Autodesk Inventor part; units mm, degrees
(part 2 of 2)
  line L161 (52.6404, 40.6164) -> (52.6404, 40.3516)
  line L162 (52.6404, 40.3516) -> (50.5162, 40.3516)
  line L163 (50.5162, 40.3516) -> (52.6404, 39.7455)
  line L164 (52.6404, 39.7455) -> (52.6404, 39.4984)
  line L165 (52.6404, 39.4984) -> (50.4789, 38.8943)
  line L166 (50.4789, 38.8943) -> (52.6404, 38.8943)
  line L167 (52.6404, 38.8943) -> (52.6404, 38.6295)
  line L168 (52.6404, 41.8638) -> (50.1004, 41.8638)
  line L169 (50.1004, 41.8638) -> (50.1004, 42.1384)
  line L170 (50.1004, 42.1384) -> (51.3596, 42.1384)
  line L171 (51.3596, 42.1384) -> (50.1004, 43.174)
  line L172 (50.1004, 43.174) -> (50.1004, 43.5487)
  line L173 (50.1004, 43.5487) -> (51.1301, 42.6739)
  line L174 (51.1301, 42.6739) -> (52.6404, 43.5859)
  line L175 (52.6404, 43.5859) -> (52.6404, 43.2211)
  line L176 (52.6404, 43.2211) -> (51.3576, 42.4797)
  line L177 (51.3576, 42.4797) -> (51.7597, 42.1384)
  line L178 (51.7597, 42.1384) -> (52.6404, 42.1384)
  line L179 (52.6404, 42.1384) -> (52.6404, 41.8638)
  line L180 (52.05, 44.8059) -> (52.0892, 45.0687)
  spline S97 degree 2 poles (52.0892, 45.0687) (52.3834, 45.0021) (52.6835, 44.6588) (52.6835, 44.4038) knots 0 0 0 1 2 2 2
  spline S98 degree 2 poles (52.6835, 44.4038) (52.6835, 44.0841) (52.1971, 43.6879) (51.7362, 43.6879) knots 0 0 0 1 2 2 2
  spline S99 degree 2 poles (51.7362, 43.6879) (51.2595, 43.6879) (50.7594, 44.088) (50.7594, 44.394) knots 0 0 0 1 2 2 2
  spline S100 degree 2 poles (50.7594, 44.394) (50.7594, 44.6863) (51.2517, 45.0785) (51.7185, 45.0785) knots 0 0 0 1 2 2 2
  line L181 (51.7185, 45.0785) -> (51.8009, 45.0766)
  line L182 (51.8009, 45.0766) -> (51.8009, 43.9507)
  spline S101 degree 2 poles (51.8009, 43.9507) (52.1108, 43.9664) (52.4266, 44.2234) (52.4266, 44.4058) knots 0 0 0 1 2 2 2
  spline S102 degree 2 poles (52.4266, 44.4058) (52.4266, 44.6941) (52.05, 44.8059) knots 0 0 0 1 1 1
  line L183 (51.5439, 43.9664) -> (51.5439, 44.8079)
  spline S103 degree 2 poles (51.5439, 44.8079) (51.3047, 44.7902) (51.187, 44.7059) knots 0 0 0 1 1 1
  spline S104 degree 2 poles (51.187, 44.7059) (51.0163, 44.5823) (51.0163, 44.3921) knots 0 0 0 1 1 1
  spline S105 degree 2 poles (51.0163, 44.3921) (51.0163, 44.2214) (51.3027, 43.9782) (51.5439, 43.9664) knots 0 0 0 1 2 2 2
  line L184 (53.3504, 45.3865) -> (53.0562, 45.359)
  spline S106 degree 2 poles (53.0562, 45.359) (53.0836, 45.4434) (53.0836, 45.5042) knots 0 0 0 1 1 1
  spline S107 degree 2 poles (53.0836, 45.5042) (53.0836, 45.5846) (53.0169, 45.6905) (52.9483, 45.7238) knots 0 0 0 1 2 2 2
  spline S108 degree 2 poles (52.9483, 45.7238) (52.9248, 45.7356) (52.6384, 45.8239) knots 0 0 0 1 1 1
  line L185 (52.6384, 45.8239) -> (50.8006, 45.2531)
  line L186 (50.8006, 45.2531) -> (50.8006, 45.5277)
  line L187 (50.8006, 45.5277) -> (51.8617, 45.8435)
  spline S109 degree 2 poles (51.8617, 45.8435) (52.0598, 45.9004) (52.2853, 45.9514) knots 0 0 0 1 1 1
  spline S110 degree 2 poles (52.2853, 45.9514) (52.0716, 45.9945) (51.8695, 46.0553) knots 0 0 0 1 1 1
  line L188 (51.8695, 46.0553) -> (50.8006, 46.377)
  line L189 (50.8006, 46.377) -> (50.8006, 46.6339)
  line L190 (50.8006, 46.6339) -> (52.6717, 46.0612)
  spline S111 degree 2 poles (52.6717, 46.0612) (53.0366, 45.9494) (53.2798, 45.82) (53.3876, 45.6552) (53.3876, 45.5512) knots 0 0 0 1 2 3 3 3
  spline S112 degree 2 poles (53.3876, 45.5512) (53.3876, 45.4787) (53.3504, 45.3865) knots 0 0 0 1 1 1
  point P0 (0, 0)
  constraints: 2 horizontal, 1 vertical, 6 other
sketch "Sketch15" plane through (0, 4.35, 0) normal (0, 1, 0) x (1, 0, 0)
  point P0 (0, 0)
sketch "Sketch16" plane through (0, 1.6, 0) normal (0, 1, 0) x (1, 0, 0)
  line L0 (10.625, 36) -> (13.125, 36)
  line L1 (13.125, 36) -> (13.125, 40.5)
  line L2 (13.125, 40.5) -> (10.625, 40.5)
  line L3 (10.625, 40.5) -> (10.625, 36)
  line L4 (23.75, 43.5) -> (32.75, 43.5) projected
  line L5 (6.5, 7.1) -> (6.5, 57.9) projected
  line L6 (17.25, 61) -> (17.25, 23) projected
  point P0 (0, 0)
  dimension "d172" = 3
  dimension "d173" = 2.5
  dimension "d174" = 4.5
  dimension "d175" = 4.125
  dimension "d176" = 4.125
  constraints: 8 end point, 2 parallel, 1 horizontal, 1 perpendicular
  measures "d172" distance between parallel lines of L4 L2
  measures "d173" distance of L1.end L2.end
  measures "d174" distance of L0.end L1.end
  measures "d175" distance between parallel lines of L5 L3
  measures "d176" distance between parallel lines of L6 L1
extrude "Extrusion17" add sketch "Sketch16" along normal blind 1
ref_plane "Work Plane1" through (13.125, 1.6, -39.6) normal (0, 0, -1) x (-1, 0, 0)
sketch "Sketch17" plane through (13.125, 1.6, -39.6) normal (0, 0, -1) x (-1, 0, 0)
  line L0 (0, 0) -> (0, 1) projected
  line L1 (0, 0.9) -> (-0.25, 0.9)
  line L2 (0, 0.8) -> (-0.25, 0.8)
  arc A0 (-0.25, 0.8) -> (-1.05, 0) centre (-0.25, 0) ccw
  arc A1 (-0.25, 0.9) -> (-1.15, 0.1) centre (-0.25, -0.0062) ccw
  line L3 (-1.05, 0) -> (-1.5, 0)
  line L4 (-1.5, 0) -> (-1.5, 0.1)
  line L5 (-1.5, 0.1) -> (-1.15, 0.1)
  line L6 (0, 0.8) -> (0, 0.9)
  point P0 (13.125, -1.6)
  dimension "d180" = 0.1
  dimension "d181" = 0.1
  dimension "d182" = 1.5
  dimension "d183" = 0.25
  dimension "d184" = 0.1
  dimension "d185" = 0.1
  constraints: 12 end point, 4 point on circle, 3 perpendicular, 2 centre point, 2 horizontal, 2 point on line, 2 tangent, 1 collinear, 1 horizontal alignment, 1 line through centre, 1 vertical alignment
  measures "d180" distance between parallel lines of L1 L2
  measures "d181" distance of L3.end L4.end
  measures "d182" distance between parallel lines of L0 L4
  measures "d183" distance of L2.start L2.end
  measures "d184" horizontal distance of L3.start L5.end
  measures "d185" distance of L0.end L1.start
extrude "Extrusion18" add sketch "Sketch17" along normal mid plane 0.25
ref_plane "Work Plane2" through (13.125, 1.6, -39.15) normal (0, 0, -1) x (-1, 0, 0)
mirror "Mirror1" about plane through (13.125, 1.6, -39.15) normal (0, 0, -1) of "Extrusion18"
ref_plane "Work Plane3" through (13.125, 1.6, -38.25) normal (0, 0, -1) x (-1, 0, 0)
mirror "Mirror2" about plane through (13.125, 1.6, -38.25) normal (0, 0, -1) of "Extrusion18", "Mirror1"
ref_plane "Work Plane4" through (11.875, 1.6, -36) normal (1, 0, 0) x (0, 0, -1)
mirror "Mirror3" about plane through (11.875, 1.6, -36) normal (1, 0, 0) of "Extrusion18", "Mirror1", "Mirror2"
sketch "Sketch18" plane through (0, 1.6, 0) normal (0, 1, 0) x (1, 0, 0)
  line L0 (6.5, 7.1) -> (6.5, 57.9) projected
  line L1 (6.5, 8.69) -> (7.5, 8.69)
  line L2 (7.5, 8.69) -> (7.5, 8.05)
  line L3 (7.5, 8.05) -> (6.5, 8.05)
  line L4 (6.5, 8.05) -> (6.5, 8.69)
  line L5 (5.55, 48.69) -> (4.91, 48.69) projected
  line L6 (4.91, 48.69) -> (4.91, 49.33) projected
  line L7 (4.91, 49.33) -> (5.55, 49.33) projected
  line L8 (5.55, 49.33) -> (5.55, 48.69) projected
  line L9 (5.55, 38.53) -> (4.91, 38.53) projected
  line L10 (4.91, 38.53) -> (4.91, 39.17) projected
  line L11 (4.91, 39.17) -> (5.55, 39.17) projected
  line L12 (5.55, 39.17) -> (5.55, 38.53) projected
  line L13 (3.09, 56.31) -> (2.45, 56.31) projected
  line L14 (2.45, 56.31) -> (2.45, 56.95) projected
  line L15 (2.45, 56.95) -> (3.09, 56.95) projected
  line L16 (3.09, 56.95) -> (3.09, 56.31) projected
  line L17 (5.55, 10.59) -> (4.91, 10.59) projected
  line L18 (4.91, 10.59) -> (4.91, 11.23) projected
  line L19 (4.91, 11.23) -> (5.55, 11.23) projected
  line L20 (5.55, 11.23) -> (5.55, 10.59) projected
  line L21 (3.09, 13.13) -> (2.45, 13.13) projected
  line L22 (2.45, 13.13) -> (2.45, 13.77) projected
  line L23 (2.45, 13.77) -> (3.09, 13.77) projected
  line L24 (3.09, 13.77) -> (3.09, 13.13) projected
  line L25 (3.09, 46.15) -> (2.45, 46.15) projected
  line L26 (2.45, 46.15) -> (2.45, 46.79) projected
  line L27 (2.45, 46.79) -> (3.09, 46.79) projected
  line L28 (3.09, 46.79) -> (3.09, 46.15) projected
  line L29 (3.09, 23.29) -> (2.45, 23.29) projected
  line L30 (2.45, 23.29) -> (2.45, 23.93) projected
  line L31 (2.45, 23.93) -> (3.09, 23.93) projected
  line L32 (3.09, 23.93) -> (3.09, 23.29) projected
  line L33 (3.09, 20.75) -> (2.45, 20.75) projected
  line L34 (2.45, 20.75) -> (2.45, 21.39) projected
  line L35 (2.45, 21.39) -> (3.09, 21.39) projected
  line L36 (3.09, 21.39) -> (3.09, 20.75) projected
  line L37 (3.09, 28.37) -> (2.45, 28.37) projected
  line L38 (2.45, 28.37) -> (2.45, 29.01) projected
  line L39 (2.45, 29.01) -> (3.09, 29.01) projected
  line L40 (3.09, 29.01) -> (3.09, 28.37) projected
  line L41 (3.09, 33.45) -> (2.45, 33.45) projected
  line L42 (2.45, 33.45) -> (2.45, 34.09) projected
  line L43 (2.45, 34.09) -> (3.09, 34.09) projected
  line L44 (3.09, 34.09) -> (3.09, 33.45) projected
  line L45 (3.09, 30.91) -> (2.45, 30.91) projected
  line L46 (2.45, 30.91) -> (2.45, 31.55) projected
  line L47 (2.45, 31.55) -> (3.09, 31.55) projected
  line L48 (3.09, 31.55) -> (3.09, 30.91) projected
  line L49 (5.55, 25.83) -> (4.91, 25.83) projected
  line L50 (4.91, 25.83) -> (4.91, 26.47) projected
  line L51 (4.91, 26.47) -> (5.55, 26.47) projected
  line L52 (5.55, 26.47) -> (5.55, 25.83) projected
  line L53 (5.55, 23.29) -> (4.91, 23.29) projected
  line L54 (4.91, 23.29) -> (4.91, 23.93) projected
  line L55 (4.91, 23.93) -> (5.55, 23.93) projected
  line L56 (5.55, 23.93) -> (5.55, 23.29) projected
  line L57 (5.55, 20.75) -> (4.91, 20.75) projected
  line L58 (4.91, 20.75) -> (4.91, 21.39) projected
  line L59 (4.91, 21.39) -> (5.55, 21.39) projected
  line L60 (5.55, 21.39) -> (5.55, 20.75) projected
  line L61 (3.09, 18.21) -> (2.45, 18.21) projected
  line L62 (2.45, 18.21) -> (2.45, 18.85) projected
  line L63 (2.45, 18.85) -> (3.09, 18.85) projected
  line L64 (3.09, 18.85) -> (3.09, 18.21) projected
  line L65 (3.09, 15.67) -> (2.45, 15.67) projected
  line L66 (2.45, 15.67) -> (2.45, 16.31) projected
  line L67 (2.45, 16.31) -> (3.09, 16.31) projected
  line L68 (3.09, 16.31) -> (3.09, 15.67) projected
  line L69 (3.09, 53.77) -> (2.45, 53.77) projected
  line L70 (2.45, 53.77) -> (2.45, 54.41) projected
  line L71 (2.45, 54.41) -> (3.09, 54.41) projected
  line L72 (3.09, 54.41) -> (3.09, 53.77) projected
  line L73 (5.55, 56.31) -> (4.91, 56.31) projected
  line L74 (4.91, 56.31) -> (4.91, 56.95) projected
  line L75 (4.91, 56.95) -> (5.55, 56.95) projected
  line L76 (5.55, 56.95) -> (5.55, 56.31) projected
  line L77 (5.55, 41.07) -> (4.91, 41.07) projected
  line L78 (4.91, 41.07) -> (4.91, 41.71) projected
  line L79 (4.91, 41.71) -> (5.55, 41.71) projected
  line L80 (5.55, 41.71) -> (5.55, 41.07) projected
  line L81 (5.55, 51.23) -> (4.91, 51.23) projected
  line L82 (4.91, 51.23) -> (4.91, 51.87) projected
  line L83 (4.91, 51.87) -> (5.55, 51.87) projected
  line L84 (5.55, 51.87) -> (5.55, 51.23) projected
  line L85 (5.55, 46.15) -> (4.91, 46.15) projected
  line L86 (4.91, 46.15) -> (4.91, 46.79) projected
  line L87 (4.91, 46.79) -> (5.55, 46.79) projected
  line L88 (5.55, 46.79) -> (5.55, 46.15) projected
  line L89 (5.55, 35.99) -> (4.91, 35.99) projected
  line L90 (4.91, 35.99) -> (4.91, 36.63) projected
  line L91 (4.91, 36.63) -> (5.55, 36.63) projected
  line L92 (5.55, 36.63) -> (5.55, 35.99) projected
  line L93 (5.55, 8.05) -> (4.91, 8.05) projected
  line L94 (4.91, 8.05) -> (4.91, 8.69) projected
  line L95 (4.91, 8.69) -> (5.55, 8.69) projected
  line L96 (5.55, 8.69) -> (5.55, 8.05) projected
  line L97 (3.09, 51.23) -> (2.45, 51.23) projected
  line L98 (2.45, 51.23) -> (2.45, 51.87) projected
  line L99 (2.45, 51.87) -> (3.09, 51.87) projected
  line L100 (3.09, 51.87) -> (3.09, 51.23) projected
  line L101 (3.09, 48.69) -> (2.45, 48.69) projected
  line L102 (2.45, 48.69) -> (2.45, 49.33) projected
  line L103 (2.45, 49.33) -> (3.09, 49.33) projected
  line L104 (3.09, 49.33) -> (3.09, 48.69) projected
  line L105 (5.55, 18.21) -> (4.91, 18.21) projected
  line L106 (4.91, 18.21) -> (4.91, 18.85) projected
  line L107 (4.91, 18.85) -> (5.55, 18.85) projected
  line L108 (5.55, 18.85) -> (5.55, 18.21) projected
  line L109 (3.09, 41.07) -> (2.45, 41.07) projected
  line L110 (2.45, 41.07) -> (2.45, 41.71) projected
  line L111 (2.45, 41.71) -> (3.09, 41.71) projected
  line L112 (3.09, 41.71) -> (3.09, 41.07) projected
  line L113 (3.09, 25.83) -> (2.45, 25.83) projected
  line L114 (2.45, 25.83) -> (2.45, 26.47) projected
  line L115 (2.45, 26.47) -> (3.09, 26.47) projected
  line L116 (3.09, 26.47) -> (3.09, 25.83) projected
  line L117 (3.09, 35.99) -> (2.45, 35.99) projected
  line L118 (2.45, 35.99) -> (2.45, 36.63) projected
  line L119 (2.45, 36.63) -> (3.09, 36.63) projected
  line L120 (3.09, 36.63) -> (3.09, 35.99) projected
  line L121 (5.55, 30.91) -> (4.91, 30.91) projected
  line L122 (4.91, 30.91) -> (4.91, 31.55) projected
  line L123 (4.91, 31.55) -> (5.55, 31.55) projected
  line L124 (5.55, 31.55) -> (5.55, 30.91) projected
  line L125 (5.55, 28.37) -> (4.91, 28.37) projected
  line L126 (4.91, 28.37) -> (4.91, 29.01) projected
  line L127 (4.91, 29.01) -> (5.55, 29.01) projected
  line L128 (5.55, 29.01) -> (5.55, 28.37) projected
  line L129 (3.09, 38.53) -> (2.45, 38.53) projected
  line L130 (2.45, 38.53) -> (2.45, 39.17) projected
  line L131 (2.45, 39.17) -> (3.09, 39.17) projected
  line L132 (3.09, 39.17) -> (3.09, 38.53) projected
  line L133 (3.09, 8.69) -> (3.09, 8.05) projected
  line L134 (3.09, 8.05) -> (2.45, 8.05) projected
  line L135 (2.45, 8.05) -> (2.45, 8.69) projected
  line L136 (2.45, 8.69) -> (3.09, 8.69) projected
  line L137 (3.09, 43.61) -> (2.45, 43.61) projected
  line L138 (2.45, 43.61) -> (2.45, 44.25) projected
  line L139 (2.45, 44.25) -> (3.09, 44.25) projected
  line L140 (3.09, 44.25) -> (3.09, 43.61) projected
  line L141 (5.55, 15.67) -> (4.91, 15.67) projected
  line L142 (4.91, 15.67) -> (4.91, 16.31) projected
  line L143 (4.91, 16.31) -> (5.55, 16.31) projected
  line L144 (5.55, 16.31) -> (5.55, 15.67) projected
  line L145 (5.55, 13.13) -> (4.91, 13.13) projected
  line L146 (4.91, 13.13) -> (4.91, 13.77) projected
  line L147 (4.91, 13.77) -> (5.55, 13.77) projected
  line L148 (5.55, 13.77) -> (5.55, 13.13) projected
  line L149 (3.09, 10.59) -> (2.45, 10.59) projected
  line L150 (2.45, 10.59) -> (2.45, 11.23) projected
  line L151 (2.45, 11.23) -> (3.09, 11.23) projected
  line L152 (3.09, 11.23) -> (3.09, 10.59) projected
  line L153 (5.55, 33.45) -> (4.91, 33.45) projected
  line L154 (4.91, 33.45) -> (4.91, 34.09) projected
  line L155 (4.91, 34.09) -> (5.55, 34.09) projected
  line L156 (5.55, 34.09) -> (5.55, 33.45) projected
  line L157 (5.55, 43.61) -> (4.91, 43.61) projected
  line L158 (4.91, 43.61) -> (4.91, 44.25) projected
  line L159 (4.91, 44.25) -> (5.55, 44.25) projected
  line L160 (5.55, 44.25) -> (5.55, 43.61) projected
  line L161 (5.55, 53.77) -> (4.91, 53.77) projected
  line L162 (4.91, 53.77) -> (4.91, 54.41) projected
  line L163 (4.91, 54.41) -> (5.55, 54.41) projected
  line L164 (5.55, 54.41) -> (5.55, 53.77) projected
  line L165 (6.5, 7.1) -> (6.5, 57.9) projected
  line L166 (6.5, 57.9) -> (1.5, 57.9) projected
  line L167 (1.5, 57.9) -> (1.5, 7.1) projected
  line L168 (1.5, 7.1) -> (6.5, 7.1) projected
  line L169 (6.5, 11.23) -> (7.5, 11.23)
  line L170 (7.5, 10.59) -> (6.5, 10.59)
  line L171 (7.5, 11.23) -> (7.5, 10.59)
  line L172 (6.5, 10.59) -> (6.5, 11.23)
  line L173 (6.5, 13.77) -> (7.5, 13.77)
  line L174 (7.5, 13.13) -> (6.5, 13.13)
  line L175 (7.5, 13.77) -> (7.5, 13.13)
  line L176 (6.5, 13.13) -> (6.5, 13.77)
  line L177 (6.5, 16.31) -> (7.5, 16.31)
  line L178 (7.5, 15.67) -> (6.5, 15.67)
  line L179 (7.5, 16.31) -> (7.5, 15.67)
  line L180 (6.5, 15.67) -> (6.5, 16.31)
  line L181 (6.5, 18.85) -> (7.5, 18.85)
  line L182 (7.5, 18.21) -> (6.5, 18.21)
  line L183 (7.5, 18.85) -> (7.5, 18.21)
  line L184 (6.5, 18.21) -> (6.5, 18.85)
  line L185 (6.5, 21.39) -> (7.5, 21.39)
  line L186 (7.5, 20.75) -> (6.5, 20.75)
  line L187 (7.5, 21.39) -> (7.5, 20.75)
  line L188 (6.5, 20.75) -> (6.5, 21.39)
  line L189 (6.5, 23.93) -> (7.5, 23.93)
  line L190 (7.5, 23.29) -> (6.5, 23.29)
  line L191 (7.5, 23.93) -> (7.5, 23.29)
  line L192 (6.5, 23.29) -> (6.5, 23.93)
  line L193 (6.5, 26.47) -> (7.5, 26.47)
  line L194 (7.5, 25.83) -> (6.5, 25.83)
  line L195 (7.5, 26.47) -> (7.5, 25.83)
  line L196 (6.5, 25.83) -> (6.5, 26.47)
  line L197 (6.5, 29.01) -> (7.5, 29.01)
  line L198 (7.5, 28.37) -> (6.5, 28.37)
  line L199 (7.5, 29.01) -> (7.5, 28.37)
  line L200 (6.5, 28.37) -> (6.5, 29.01)
  line L201 (6.5, 31.55) -> (7.5, 31.55)
  line L202 (7.5, 30.91) -> (6.5, 30.91)
  line L203 (7.5, 31.55) -> (7.5, 30.91)
  line L204 (6.5, 30.91) -> (6.5, 31.55)
  line L205 (6.5, 34.09) -> (7.5, 34.09)
  line L206 (7.5, 33.45) -> (6.5, 33.45)
  line L207 (7.5, 34.09) -> (7.5, 33.45)
  line L208 (6.5, 33.45) -> (6.5, 34.09)
  line L209 (6.5, 36.63) -> (7.5, 36.63)
  line L210 (7.5, 35.99) -> (6.5, 35.99)
  line L211 (7.5, 36.63) -> (7.5, 35.99)
  line L212 (6.5, 35.99) -> (6.5, 36.63)
  line L213 (6.5, 39.17) -> (7.5, 39.17)
  line L214 (7.5, 38.53) -> (6.5, 38.53)
  line L215 (7.5, 39.17) -> (7.5, 38.53)
  line L216 (6.5, 38.53) -> (6.5, 39.17)
  line L217 (6.5, 41.71) -> (7.5, 41.71)
  line L218 (7.5, 41.07) -> (6.5, 41.07)
  line L219 (7.5, 41.71) -> (7.5, 41.07)
  line L220 (6.5, 41.07) -> (6.5, 41.71)
  line L221 (6.5, 44.25) -> (7.5, 44.25)
  line L222 (7.5, 43.61) -> (6.5, 43.61)
  line L223 (7.5, 44.25) -> (7.5, 43.61)
  line L224 (6.5, 43.61) -> (6.5, 44.25)
  line L225 (6.5, 46.79) -> (7.5, 46.79)
  line L226 (7.5, 46.15) -> (6.5, 46.15)
  line L227 (7.5, 46.79) -> (7.5, 46.15)
  line L228 (6.5, 46.15) -> (6.5, 46.79)
  line L229 (6.5, 49.33) -> (7.5, 49.33)
  line L230 (7.5, 48.69) -> (6.5, 48.69)
  line L231 (7.5, 49.33) -> (7.5, 48.69)
  line L232 (6.5, 48.69) -> (6.5, 49.33)
  line L233 (6.5, 51.87) -> (7.5, 51.87)
  line L234 (7.5, 51.23) -> (6.5, 51.23)
  line L235 (7.5, 51.87) -> (7.5, 51.23)
  line L236 (6.5, 51.23) -> (6.5, 51.87)
  line L237 (6.5, 54.41) -> (7.5, 54.41)
  line L238 (7.5, 53.77) -> (6.5, 53.77)
  line L239 (7.5, 54.41) -> (7.5, 53.77)
  line L240 (6.5, 53.77) -> (6.5, 54.41)
  line L241 (6.5, 56.95) -> (7.5, 56.95)
  line L242 (7.5, 56.31) -> (6.5, 56.31)
  line L243 (7.5, 56.95) -> (7.5, 56.31)
  line L244 (6.5, 56.31) -> (6.5, 56.95)
  point P0 (0, 0)
  point P1 (6.5, 56.95)
  point P2 (6.5, 56.31)
  point P3 (6.5, 54.41)
  point P4 (6.5, 53.77)
  point P5 (6.5, 51.87)
  point P6 (6.5, 51.23)
  point P7 (6.5, 49.33)
  point P8 (6.5, 48.69)
  point P9 (6.5, 46.79)
  point P10 (6.5, 46.15)
  point P11 (6.5, 44.25)
  point P12 (6.5, 43.61)
  point P13 (6.5, 41.71)
  point P14 (6.5, 41.07)
  point P15 (6.5, 39.17)
  point P16 (6.5, 38.53)
  point P17 (6.5, 36.63)
  point P18 (6.5, 35.99)
  point P19 (6.5, 34.09)
  point P20 (6.5, 33.45)
  point P21 (6.5, 31.55)
  point P22 (6.5, 30.91)
  point P23 (6.5, 29.01)
  point P24 (6.5, 28.37)
  point P25 (6.5, 26.47)
  point P26 (6.5, 25.83)
  point P27 (6.5, 23.93)
  point P28 (6.5, 23.29)
  point P29 (6.5, 21.39)
  point P30 (6.5, 20.75)
  point P31 (6.5, 18.85)
  point P32 (6.5, 18.21)
  point P33 (6.5, 16.31)
  point P34 (6.5, 15.67)
  point P35 (6.5, 13.77)
  point P36 (6.5, 13.13)
  point P37 (6.5, 11.23)
  dimension "d190" = 1
  dimension "d193" = 2.54
  constraints: 160 end point, 76 vertical alignment, 40 parallel, 38 collinear, 3 horizontal alignment, 1 horizontal, 1 perpendicular, 1 point on line, 2 other
  measures "d190" distance of L2.end L3.end
  measures "d193" distance of L1.start L169.start
extrude "Extrusion19" add sketch "Sketch18" along normal blind 0.25 contours L0 L1 L2 L3 | L0 L169 L171 L170 | L241 L243 L242 L0 | L0 L173 L175 L174 | L237 L239 L238 L0 | L0 L177 L179 L178 | L233 L235 L234 L0 | L0 L181 L183 L182 | L229 L231 L230 L0 | L0 L185 L187 L186 | L225 L227 L226 L0 | L0 L189 L191 L190 | L221 L223 L222 L0 | L0 L193 L195 L194 | L217 L219 L218 L0 | L0 L197 L199 L198 | L213 L215 L214 L0 | L0 L201 L203 L202 | L209 L211 L210 L0 | L0 L205 L207 L206
ref_plane "Work Plane5" through (4, 1.6, -57.9) normal (1, 0, 0) x (0, 0, -1)
mirror "Mirror4" about plane through (4, 1.6, -57.9) normal (1, 0, 0) of "Extrusion19"
extrude "Extrusion20" add sketch "Sketch14" along normal blind 0.01
sketch "Sketch19" plane through (0, 0, 0) normal (0, -1, 0) x (1, 0, 0)
  circle A0 centre (53, -3.5) radius 3 projected
  circle A1 centre (4, -3.5) radius 3 projected
  circle A2 centre (53, -61.5) radius 3 projected
  circle A3 centre (4, -61.5) radius 3 projected
  point P0 (0, 0)
extrude "Extrusion21" cut sketch "Sketch19" against normal blind 0.02
sketch "Sketch20" plane through (0, 0, 0) normal (0, -1, 0) x (1, 0, 0)
  line L0 (5.55, -48.69) -> (4.91, -48.69) projected
  line L1 (4.91, -48.69) -> (4.91, -49.33) projected
  line L2 (4.91, -49.33) -> (5.55, -49.33) projected
  line L3 (5.55, -49.33) -> (5.55, -48.69) projected
  line L4 (5.55, -38.53) -> (4.91, -38.53) projected
  line L5 (4.91, -38.53) -> (4.91, -39.17) projected
  line L6 (4.91, -39.17) -> (5.55, -39.17) projected
  line L7 (5.55, -39.17) -> (5.55, -38.53) projected
  line L8 (3.09, -56.31) -> (2.45, -56.31) projected
  line L9 (2.45, -56.31) -> (2.45, -56.95) projected
  line L10 (2.45, -56.95) -> (3.09, -56.95) projected
  line L11 (3.09, -56.95) -> (3.09, -56.31) projected
  line L12 (5.55, -10.59) -> (4.91, -10.59) projected
  line L13 (4.91, -10.59) -> (4.91, -11.23) projected
  line L14 (4.91, -11.23) -> (5.55, -11.23) projected
  line L15 (5.55, -11.23) -> (5.55, -10.59) projected
  line L16 (3.09, -13.13) -> (2.45, -13.13) projected
  line L17 (2.45, -13.13) -> (2.45, -13.77) projected
  line L18 (2.45, -13.77) -> (3.09, -13.77) projected
  line L19 (3.09, -13.77) -> (3.09, -13.13) projected
  line L20 (3.09, -46.15) -> (2.45, -46.15) projected
  line L21 (2.45, -46.15) -> (2.45, -46.79) projected
  line L22 (2.45, -46.79) -> (3.09, -46.79) projected
  line L23 (3.09, -46.79) -> (3.09, -46.15) projected
  line L24 (3.09, -23.29) -> (2.45, -23.29) projected
  line L25 (2.45, -23.29) -> (2.45, -23.93) projected
  line L26 (2.45, -23.93) -> (3.09, -23.93) projected
  line L27 (3.09, -23.93) -> (3.09, -23.29) projected
  line L28 (3.09, -20.75) -> (2.45, -20.75) projected
  line L29 (2.45, -20.75) -> (2.45, -21.39) projected
  line L30 (2.45, -21.39) -> (3.09, -21.39) projected
  line L31 (3.09, -21.39) -> (3.09, -20.75) projected
  line L32 (3.09, -28.37) -> (2.45, -28.37) projected
  line L33 (2.45, -28.37) -> (2.45, -29.01) projected
  line L34 (2.45, -29.01) -> (3.09, -29.01) projected
  line L35 (3.09, -29.01) -> (3.09, -28.37) projected
  line L36 (3.09, -33.45) -> (2.45, -33.45) projected
  line L37 (2.45, -33.45) -> (2.45, -34.09) projected
  line L38 (2.45, -34.09) -> (3.09, -34.09) projected
  line L39 (3.09, -34.09) -> (3.09, -33.45) projected
  line L40 (3.09, -30.91) -> (2.45, -30.91) projected
  line L41 (2.45, -30.91) -> (2.45, -31.55) projected
  line L42 (2.45, -31.55) -> (3.09, -31.55) projected
  line L43 (3.09, -31.55) -> (3.09, -30.91) projected
  line L44 (5.55, -25.83) -> (4.91, -25.83) projected
  line L45 (4.91, -25.83) -> (4.91, -26.47) projected
  line L46 (4.91, -26.47) -> (5.55, -26.47) projected
  line L47 (5.55, -26.47) -> (5.55, -25.83) projected
  line L48 (5.55, -23.29) -> (4.91, -23.29) projected
  line L49 (4.91, -23.29) -> (4.91, -23.93) projected
  line L50 (4.91, -23.93) -> (5.55, -23.93) projected
  line L51 (5.55, -23.93) -> (5.55, -23.29) projected
  line L52 (5.55, -20.75) -> (4.91, -20.75) projected
  line L53 (4.91, -20.75) -> (4.91, -21.39) projected
  line L54 (4.91, -21.39) -> (5.55, -21.39) projected
  line L55 (5.55, -21.39) -> (5.55, -20.75) projected
  line L56 (3.09, -18.21) -> (2.45, -18.21) projected
  line L57 (2.45, -18.21) -> (2.45, -18.85) projected
  line L58 (2.45, -18.85) -> (3.09, -18.85) projected
  line L59 (3.09, -18.85) -> (3.09, -18.21) projected
  line L60 (3.09, -15.67) -> (2.45, -15.67) projected
  line L61 (2.45, -15.67) -> (2.45, -16.31) projected
  line L62 (2.45, -16.31) -> (3.09, -16.31) projected
  line L63 (3.09, -16.31) -> (3.09, -15.67) projected
  line L64 (3.09, -53.77) -> (2.45, -53.77) projected
  line L65 (2.45, -53.77) -> (2.45, -54.41) projected
  line L66 (2.45, -54.41) -> (3.09, -54.41) projected
  line L67 (3.09, -54.41) -> (3.09, -53.77) projected
  line L68 (5.55, -56.31) -> (4.91, -56.31) projected
  line L69 (4.91, -56.31) -> (4.91, -56.95) projected
  line L70 (4.91, -56.95) -> (5.55, -56.95) projected
  line L71 (5.55, -56.95) -> (5.55, -56.31) projected
  line L72 (5.55, -41.07) -> (4.91, -41.07) projected
  line L73 (4.91, -41.07) -> (4.91, -41.71) projected
  line L74 (4.91, -41.71) -> (5.55, -41.71) projected
  line L75 (5.55, -41.71) -> (5.55, -41.07) projected
  line L76 (5.55, -51.23) -> (4.91, -51.23) projected
  line L77 (4.91, -51.23) -> (4.91, -51.87) projected
  line L78 (4.91, -51.87) -> (5.55, -51.87) projected
  line L79 (5.55, -51.87) -> (5.55, -51.23) projected
  line L80 (5.55, -46.15) -> (4.91, -46.15) projected
  line L81 (4.91, -46.15) -> (4.91, -46.79) projected
  line L82 (4.91, -46.79) -> (5.55, -46.79) projected
  line L83 (5.55, -46.79) -> (5.55, -46.15) projected
  line L84 (5.55, -35.99) -> (4.91, -35.99) projected
  line L85 (4.91, -35.99) -> (4.91, -36.63) projected
  line L86 (4.91, -36.63) -> (5.55, -36.63) projected
  line L87 (5.55, -36.63) -> (5.55, -35.99) projected
  line L88 (5.55, -8.05) -> (4.91, -8.05) projected
  line L89 (4.91, -8.05) -> (4.91, -8.69) projected
  line L90 (4.91, -8.69) -> (5.55, -8.69) projected
  line L91 (5.55, -8.69) -> (5.55, -8.05) projected
  line L92 (3.09, -51.23) -> (2.45, -51.23) projected
  line L93 (2.45, -51.23) -> (2.45, -51.87) projected
  line L94 (2.45, -51.87) -> (3.09, -51.87) projected
  line L95 (3.09, -51.87) -> (3.09, -51.23) projected
  line L96 (3.09, -48.69) -> (2.45, -48.69) projected
  line L97 (2.45, -48.69) -> (2.45, -49.33) projected
  line L98 (2.45, -49.33) -> (3.09, -49.33) projected
  line L99 (3.09, -49.33) -> (3.09, -48.69) projected
  line L100 (5.55, -18.21) -> (4.91, -18.21) projected
  line L101 (4.91, -18.21) -> (4.91, -18.85) projected
  line L102 (4.91, -18.85) -> (5.55, -18.85) projected
  line L103 (5.55, -18.85) -> (5.55, -18.21) projected
  line L104 (3.09, -41.07) -> (2.45, -41.07) projected
  line L105 (2.45, -41.07) -> (2.45, -41.71) projected
  line L106 (2.45, -41.71) -> (3.09, -41.71) projected
  line L107 (3.09, -41.71) -> (3.09, -41.07) projected
  line L108 (3.09, -25.83) -> (2.45, -25.83) projected
  line L109 (2.45, -25.83) -> (2.45, -26.47) projected
  line L110 (2.45, -26.47) -> (3.09, -26.47) projected
  line L111 (3.09, -26.47) -> (3.09, -25.83) projected
  line L112 (3.09, -35.99) -> (2.45, -35.99) projected
  line L113 (2.45, -35.99) -> (2.45, -36.63) projected
  line L114 (2.45, -36.63) -> (3.09, -36.63) projected
  line L115 (3.09, -36.63) -> (3.09, -35.99) projected
  line L116 (5.55, -30.91) -> (4.91, -30.91) projected
  line L117 (4.91, -30.91) -> (4.91, -31.55) projected
  line L118 (4.91, -31.55) -> (5.55, -31.55) projected
  line L119 (5.55, -31.55) -> (5.55, -30.91) projected
  line L120 (5.55, -28.37) -> (4.91, -28.37) projected
  line L121 (4.91, -28.37) -> (4.91, -29.01) projected
  line L122 (4.91, -29.01) -> (5.55, -29.01) projected
  line L123 (5.55, -29.01) -> (5.55, -28.37) projected
  line L124 (3.09, -38.53) -> (2.45, -38.53) projected
  line L125 (2.45, -38.53) -> (2.45, -39.17) projected
  line L126 (2.45, -39.17) -> (3.09, -39.17) projected
  line L127 (3.09, -39.17) -> (3.09, -38.53) projected
  line L128 (3.09, -8.69) -> (3.09, -8.05) projected
  line L129 (3.09, -8.05) -> (2.45, -8.05) projected
  line L130 (2.45, -8.05) -> (2.45, -8.69) projected
  line L131 (2.45, -8.69) -> (3.09, -8.69) projected
  line L132 (3.09, -43.61) -> (2.45, -43.61) projected
  line L133 (2.45, -43.61) -> (2.45, -44.25) projected
  line L134 (2.45, -44.25) -> (3.09, -44.25) projected
  line L135 (3.09, -44.25) -> (3.09, -43.61) projected
  line L136 (5.55, -15.67) -> (4.91, -15.67) projected
  line L137 (4.91, -15.67) -> (4.91, -16.31) projected
  line L138 (4.91, -16.31) -> (5.55, -16.31) projected
  line L139 (5.55, -16.31) -> (5.55, -15.67) projected
  line L140 (5.55, -13.13) -> (4.91, -13.13) projected
  line L141 (4.91, -13.13) -> (4.91, -13.77) projected
  line L142 (4.91, -13.77) -> (5.55, -13.77) projected
  line L143 (5.55, -13.77) -> (5.55, -13.13) projected
  line L144 (3.09, -10.59) -> (2.45, -10.59) projected
  line L145 (2.45, -10.59) -> (2.45, -11.23) projected
  line L146 (2.45, -11.23) -> (3.09, -11.23) projected
  line L147 (3.09, -11.23) -> (3.09, -10.59) projected
  line L148 (5.55, -33.45) -> (4.91, -33.45) projected
  line L149 (4.91, -33.45) -> (4.91, -34.09) projected
  line L150 (4.91, -34.09) -> (5.55, -34.09) projected
  line L151 (5.55, -34.09) -> (5.55, -33.45) projected
  line L152 (5.55, -43.61) -> (4.91, -43.61) projected
  line L153 (4.91, -43.61) -> (4.91, -44.25) projected
  line L154 (4.91, -44.25) -> (5.55, -44.25) projected
  line L155 (5.55, -44.25) -> (5.55, -43.61) projected
  line L156 (5.55, -53.77) -> (4.91, -53.77) projected
  line L157 (4.91, -53.77) -> (4.91, -54.41) projected
  line L158 (4.91, -54.41) -> (5.55, -54.41) projected
  line L159 (5.55, -54.41) -> (5.55, -53.77) projected
  line L160 (6.5, -7.1) -> (6.5, -57.9) projected
  line L161 (6.5, -57.9) -> (1.5, -57.9) projected
  line L162 (1.5, -57.9) -> (1.5, -7.1) projected
  line L163 (1.5, -7.1) -> (6.5, -7.1) projected
  point P0 (0, 0)
extrude "Extrusion22" cut sketch "Sketch20" against normal through all contours L3 L2 L1 L0 | L7 L6 L5 L4 | L11 L10 L9 L8 | L15 L14 L13 L12 | L19 L18 L17 L16 | L23 L22 L21 L20 | L27 L26 L25 L24 | L31 L30 L29 L28 | L35 L34 L33 L32 | L39 L38 L37 L36 | L43 L42 L41 L40 | L47 L46 L45 L44 | L51 L50 L49 L48 | L55 L54 L53 L52 | L59 L58 L57 L56 | L63 L62 L61 L60 | L67 L66 L65 L64 | L71 L70 L69 L68 | L75 L74 L73 L72 | L79 L78 L77 L76 | L83 L82 L81 L80 | L87 L86 L85 L84 | L91 L90 L89 L88 | L95 L94 L93 L92 | L99 L98 L97 L96 | L103 L102 L101 L100 | L107 L106 L105 L104 | L111 L110 L109 L108 | L115 L114 L113 L112 | L119 L118 L117 L116 | L123 L122 L121 L120 | L127 L126 L125 L124 | L131 L130 L129 L128 | L135 L134 L133 L132 | L139 L138 L137 L136 | L143 L142 L141 L140 | L147 L146 L145 L144 | L151 L150 L149 L148 | L155 L154 L153 L152 | L159 L158 L157 L156
extrude "Extrusion23" add sketch "Sketch11" along normal blind 1.9 contours L0 L7 L2 L8
sketch "Sketch21" plane through (0, 1.6, 0) normal (0, 1, 0) x (1, 0, 0)
  line L0 (45.3625, 29.5277) -> (48.4125, 29.5277)
  line L1 (48.9125, 30.0277) -> (48.9125, 45.7978)
  line L2 (48.4125, 46.2978) -> (45.3625, 46.2978)
  line L3 (44.8625, 45.7978) -> (44.8625, 30.0277)
  arc A0 (44.8625, 30.0277) -> (45.3625, 29.5277) centre (45.3625, 30.0277) ccw
  arc A1 (48.4125, 29.5277) -> (48.9125, 30.0277) centre (48.4125, 30.0277) ccw
  arc A2 (48.9125, 45.7978) -> (48.4125, 46.2978) centre (48.4125, 45.7978) ccw
  arc A3 (45.3625, 46.2978) -> (44.8625, 45.7978) centre (45.3625, 45.7978) ccw
  line L4 (44.6125, 30.0277) -> (44.6125, 45.7978)
  arc A4 (45.3625, 46.5478) -> (44.6125, 45.7978) centre (45.3625, 45.7978) ccw
  line L5 (45.3625, 46.5478) -> (48.4125, 46.5478)
  arc A5 (49.1625, 45.7978) -> (48.4125, 46.5478) centre (48.4125, 45.7978) ccw
  line L6 (49.1625, 45.7978) -> (49.1625, 30.0277)
  arc A6 (48.4125, 29.2777) -> (49.1625, 30.0277) centre (48.4125, 30.0277) ccw
  line L7 (48.4125, 29.2777) -> (45.3625, 29.2777)
  arc A7 (44.6125, 30.0277) -> (45.3625, 29.2777) centre (45.3625, 30.0277) ccw
  line L8 (55.5, 47.5) -> (41, 47.5) projected
  line L9 (56.5, 3.5) -> (56.5, 46.5) projected
  line L10 (48.4125, 42.5313) -> (48.4125, 42.861) projected
  line L11 (45.3625, 43.69) -> (45.3625, 41.707) projected
  line L12 (45.3625, 30.2277) -> (48.4125, 30.2277) projected
  line L13 (47.0841, 45.5978) -> (46.7356, 45.5978) projected
  point P0 (0, 0)
  dimension "d211" = 0.5
  dimension "d212" = 0.25
  dimension "d215" = 0.5
  dimension "d216" = 0.5
  dimension "d217" = 0.7
  dimension "d218" = 0.7
  constraints: 16 end point, 16 point on circle, 8 centre point, 8 tangent, 4 parallel, 3 equal radius, 2 perpendicular, 1 horizontal, 7 other
  measures "d211" radius of A0
  measures "d212" distance between parallel lines of L4 L3
  measures "d215" distance between parallel lines of L10 L1
  measures "d216" distance between parallel lines of L3 L11
  measures "d217" distance between parallel lines of L0 L12
  measures "d218" distance between parallel lines of L13 L2
extrude "Extrusion24" add sketch "Sketch21" along normal up to surface (0.01 mm away)
sketch "Sketch22" plane through (0, 4.35, 0) normal (0, 1, 0) x (1, 0, 0)
  line L0 (30.75, 34.6545) -> (25.75, 34.6545) construction
  line L1 (25.75, 34.6545) -> (25.75, 37.1545) construction
  line L2 (25.75, 37.1545) -> (30.75, 37.1545) construction
  line L3 (30.75, 37.1545) -> (30.75, 34.6545) construction
  line L4 (26.4257, 37.1545) -> (31.4257, 37.1545) construction
  line L5 (31.4257, 37.1545) -> (31.4257, 34.6545) construction
  line L6 (31.4257, 34.6545) -> (26.4257, 34.6545) construction
  line L7 (26.4257, 34.6545) -> (26.4257, 37.1545) construction
  line L8 (23.4045, 33.5) -> (23.4045, 42.5) projected
  line L9 (33.0955, 42.5) -> (33.0955, 33.5) projected
  line L10 (32.75, 33.1545) -> (23.75, 33.1545) projected
  line L11 (30.4788, 36.3941) -> (30.4788, 35.3941)
  line L12 (30.4788, 35.3941) -> (30.3202, 35.3941)
  line L13 (30.3202, 35.3941) -> (30.3202, 35.805)
  line L14 (30.3202, 35.805) -> (29.6975, 35.805)
  line L15 (29.6975, 35.805) -> (29.6975, 35.3941)
  line L16 (29.6975, 35.3941) -> (29.539, 35.3941)
  line L17 (29.539, 35.3941) -> (29.539, 36.3941)
  line L18 (29.539, 36.3941) -> (29.6975, 36.3941)
  line L19 (29.6975, 36.3941) -> (29.6975, 35.9231)
  line L20 (29.6975, 35.9231) -> (30.3202, 35.9231)
  line L21 (30.3202, 35.9231) -> (30.3202, 36.3941)
  line L22 (30.3202, 36.3941) -> (30.4788, 36.3941)
  line L23 (28.318, 36.3941) -> (28.318, 35.3941)
  line L24 (28.318, 35.3941) -> (28.1594, 35.3941)
  line L25 (28.1594, 35.3941) -> (28.1594, 36.3941)
  line L26 (28.1594, 36.3941) -> (28.318, 36.3941)
  line L27 (27.8865, 36.3941) -> (27.8865, 35.3941)
  line L28 (27.8865, 35.3941) -> (27.728, 35.3941)
  line L29 (27.728, 35.3941) -> (27.728, 36.276)
  line L30 (27.728, 36.276) -> (27.1373, 36.276)
  line L31 (27.1373, 36.276) -> (27.1373, 36.3941)
  line L32 (27.1373, 36.3941) -> (27.8865, 36.3941)
  line L33 (26.0347, 36.4149) -> (26.9286, 36.4149)
  line L34 (26.9286, 36.4149) -> (26.9286, 35.4058)
  line L35 (26.9286, 35.4058) -> (26.0347, 35.4058)
  line L36 (26.0347, 35.4058) -> (26.0347, 36.4149)
  line L37 (26.1409, 36.3311) -> (26.1409, 35.4895)
  line L38 (26.1409, 35.4895) -> (26.8225, 35.4895)
  line L39 (26.8225, 35.4895) -> (26.8225, 36.3311)
  line L40 (26.8225, 36.3311) -> (26.1409, 36.3311)
  line L41 (28.846, 35.4045) -> (28.4207, 36.4045)
  line L42 (28.4207, 36.4045) -> (28.5777, 36.4045)
  line L43 (28.5777, 36.4045) -> (28.8636, 35.6781)
  spline S0 degree 2 poles (28.8636, 35.6781) (28.8979, 35.5912) (28.9215, 35.515) knots 0 0 0 1 1 1
  spline S1 degree 2 poles (28.9215, 35.515) (28.9466, 35.5966) (28.9802, 35.6781) knots 0 0 0 1 1 1
  line L44 (28.9802, 35.6781) -> (29.2774, 36.4045)
  line L45 (29.2774, 36.4045) -> (29.4261, 36.4045)
  line L46 (29.4261, 36.4045) -> (28.9962, 35.4045)
  line L47 (28.9962, 35.4045) -> (28.846, 35.4045)
  point P0 (0, 0)
  dimension "d221" = 5
  dimension "d222" = 2.5
  dimension "d223" = 5
  dimension "d224" = 2.5
  dimension "d225" = 2.3455
  dimension "d226" = 2.3455
  dimension "d227" = 1.5
  constraints: 2 horizontal, 1 horizontal alignment, 4 other
  measures "d221" distance of L0.start L0.end
  measures "d222" distance of L2.end L0.start
  measures "d223" distance of L5.end L6.end
  measures "d224" distance of L4.end L5.end
  measures "d225" distance between parallel lines of L8 L1
  measures "d226" distance between parallel lines of L9 L3
  measures "d227" distance between parallel lines of L10 L0
extrude "Extrusion25" cut sketch "Sketch22" against normal blind 0.1
fillet "Fillet7" radius 0.05 8 edges at (26.0347, 4.3, -35.4058) (26.9286, 4.3, -35.4058) (26.8225, 4.3, -35.4895) (26.1409, 4.3, -35.4895) (26.1409, 4.3, -36.3311) (26.8225, 4.3, -36.3311) (26.9286, 4.3, -36.4149) (26.0347, 4.3, -36.4149)
ref_plane "Work Plane6" through (26.5, 1.6, -12.5) normal (1, 0, 0) x (0, 0, -1)
sketch "Sketch23" plane through (26.5, 1.6, -12.5) normal (1, 0, 0) x (0, 0, -1)
  line L0 (-3.5, 1.9) -> (-3.5, 0.5) projected
  line L1 (-3.5, 0.5) -> (-3.5, 1.9) projected
  line L2 (-3.5, 1.9) -> (-3.5, 0.5) projected
  arc A0 (-9.255, 3.1279) -> (-12.8811, -3.2509) centre (-9.7947, -0.7854) ccw
  arc A1 (-9.255, -13.6) -> (-12.8811, -3.2509) centre (-25.8366, -13.6) ccw
  line L3 (-12.5, -1.6) -> (-12.5, 0) projected
  line L4 (-9, -1.6) -> (34, -1.6) projected
  line L5 (-9.255, -13.6) -> (-4.255, -13.6) construction
  line L6 (-3.5, 0) -> (-3.5, 2.25) projected
  arc A2 (-3.5, 1.8) -> (-9.255, 3.1279) centre (-13.7578, -29.522) ccw
  line L7 (-9, 0) -> (34, 0) projected
  dimension "d232" = 3.245
  dimension "d233" = 12
  dimension "d234" = 5
  dimension "d240" = 0.1
  dimension "d241" = 5.755
  dimension "d242" = 6.3788
  dimension "d243" = 3.6261
  dimension "d244" = 3.1279
  constraints: 6 point on circle, 3 centre point, 2 end point, 2 tangent, 1 horizontal, 1 line through centre, 1 point on line
  measures "d232" distance from line of L3 L5.start
  measures "d233" distance from line of L4 L5.start
  measures "d234" distance of L5.start L5.end
  measures "d240" distance of L0.start A2.start
  measures "d241" distance from line of L0 A0.start
  measures "d242" vertical distance of A0.end A0.start
  measures "d243" horizontal distance of L5.start A0.end
  measures "d244" distance from line of L7 A0.start
sketch "Sketch24" plane through (22.55, 3.5, -9) normal (0, 0, 1) x (1, 0, 0)
  line L0 (1.45, -0.1) -> (6.45, -0.1)
  line L1 (6.45, -0.1) -> (6.45, -0.2)
  line L2 (6.45, -0.2) -> (1.45, -0.2)
  line L3 (1.45, -0.2) -> (1.45, -0.1)
  line L4 (0, 0) -> (7.9, 0) projected
  point P0 (-22.55, -3.5)
  point P1 (3.95, -0.1)
  point P2 (3.95, 0)
  dimension "d235" = 0.1
  dimension "d236" = 5
  dimension "d237" = 0.1
  constraints: 8 end point, 2 midpoint, 2 parallel, 1 horizontal, 1 perpendicular, 1 vertical alignment
  measures "d235" distance between parallel lines of L4 L0
  measures "d236" distance of L1.end L2.end
  measures "d237" distance of L0.end L1.end
sweep "Sweep2" add profiles "Sketch24" path "Sketch23" path curves A2 A0 A1
sketch "Sketch25" plane through (0, 4.35, 0) normal (0, 1, 0) x (1, 0, 0)
  line L0 (21.25, 31) -> (35.25, 31)
  line L1 (35.25, 31) -> (35.25, 45)
  line L2 (35.25, 45) -> (21.25, 45)
  line L3 (21.25, 45) -> (21.25, 31)
  line L4 (35.5, 46) -> (21, 46) projected
  line L5 (20.25, 45.25) -> (20.25, 30.75) projected
  line L6 (21, 30) -> (35.5, 30) projected
  line L7 (36.25, 30.75) -> (36.25, 45.25) projected
  point P0 (0, 0)
  dimension "d247" = 14
  dimension "d248" = 14
  dimension "d249" = 1
  dimension "d251" = 1
  dimension "d252" = 1
  dimension "d253" = 1
  constraints: 8 end point, 2 parallel, 1 horizontal, 1 perpendicular
  measures "d247" distance of L0.end L1.end
  measures "d248" distance of L1.end L2.end
  measures "d249" distance between parallel lines of L4 L2
  measures "d251" distance between parallel lines of L5 L3
  measures "d252" distance between parallel lines of L6 L0
  measures "d253" distance between parallel lines of L7 L1
extrude "Extrusion26" add sketch "Sketch25" along normal blind 1
sketch "Sketch26" plane through (0, 5.35, 0) normal (0, 1, 0) x (1, 0, 0)
  line L0 (35.25, 31) -> (35.25, 45) projected
  line L1 (35.25, 45) -> (21.25, 45) projected
  line L2 (35.25, 31) -> (34.25, 31)
  line L3 (34.25, 31) -> (34.25, 45)
  line L4 (34.25, 45) -> (35.25, 45)
  line L5 (35.25, 45) -> (35.25, 31)
  line L6 (32.0833, 31) -> (32.0833, 45)
  line L7 (33.0833, 45) -> (33.0833, 31)
  line L8 (33.0833, 31) -> (32.0833, 31)
  line L9 (32.0833, 45) -> (33.0833, 45)
  line L10 (29.9167, 31) -> (29.9167, 45)
  line L11 (30.9167, 45) -> (30.9167, 31)
  line L12 (30.9167, 31) -> (29.9167, 31)
  line L13 (29.9167, 45) -> (30.9167, 45)
  line L14 (27.75, 31) -> (27.75, 45)
  line L15 (28.75, 45) -> (28.75, 31)
  line L16 (28.75, 31) -> (27.75, 31)
  line L17 (27.75, 45) -> (28.75, 45)
  line L18 (25.5833, 31) -> (25.5833, 45)
  line L19 (26.5833, 45) -> (26.5833, 31)
  line L20 (26.5833, 31) -> (25.5833, 31)
  line L21 (25.5833, 45) -> (26.5833, 45)
  line L22 (23.4167, 31) -> (23.4167, 45)
  line L23 (24.4167, 45) -> (24.4167, 31)
  line L24 (24.4167, 31) -> (23.4167, 31)
  line L25 (23.4167, 45) -> (24.4167, 45)
  line L26 (21.25, 31) -> (21.25, 45)
  line L27 (22.25, 45) -> (22.25, 31)
  line L28 (22.25, 31) -> (21.25, 31)
  line L29 (21.25, 45) -> (22.25, 45)
  line L30 (21.25, 45) -> (21.25, 31) projected
  point P0 (0, 0)
  dimension "d256" = 1
  dimension "d259" = 2.1667
  dimension "d264" = 0
  constraints: 56 end point, 2 horizontal, 2 parallel, 1 perpendicular, 1 point on line, 48 other
  measures "d256" distance between parallel lines of L0 L3
  measures "d259" distance of L2.end L6.start
  measures "d264" distance between parallel lines of L30 L26
extrude "Extrusion27" add sketch "Sketch26" along normal blind 4
thread "Thread1"
equation "\"d82\" = d83"
equation "\"d80\" = d79"
body "Solid1"
